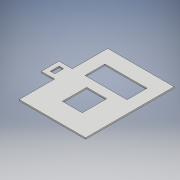
# Autodesk Inventor part: depan
Saved by Autodesk Inventor 2017 (Build 210142000, 142)
## iProperties
Created: 2017-01-06
Part Number: depan
Material: Generic
Document SubType Name: Modeling
Designer: Ghesa Bhakti
Density: 1 g/cm^3
Appearance: Default
Author: Ghesa Bhakti
Autodesk Inventor part; units mm, degrees
ref_plane "YZ Plane" through (0, 0, 0) normal (1, 0, 0) x (0, 1, 0)
ref_plane "XZ Plane" through (0, 0, 0) normal (0, 1, 0) x (-1, 0, 0)
ref_plane "XY Plane" through (0, 0, 0) normal (0, 0, 1) x (1, 0, 0)
sketch "Sketch1" plane through (0, 0, 0) normal (0, 0, 1) x (1, 0, 0)
  line L0 (27.5, 166.3577) -> (122.5, 166.3577)
  line L1 (122.5, 166.3577) -> (122.5, 121.3577)
  line L2 (122.5, 121.3577) -> (27.5, 121.3577)
  line L3 (27.5, 121.3577) -> (27.5, 166.3577)
  line L4 (52.5, 100.1) -> (97.5, 100.1)
  line L5 (97.5, 100.1) -> (97.5, 45.1)
  line L6 (97.5, 45.1) -> (52.5, 45.1)
  line L7 (52.5, 45.1) -> (52.5, 100.1)
  line L8 (0, 0) -> (150, 0)
  line L9 (0, 200) -> (150, 200)
  line L10 (0, 153.4) -> (0, 120)
  line L11 (0, 80) -> (0, 0)
  line L12 (0, 153.4) -> (0, 200)
  line L13 (0, 120) -> (-30, 120)
  line L14 (-30, 120) -> (-30, 80)
  line L15 (-30, 80) -> (0, 80)
  line L16 (-20, 110) -> (-10, 110)
  line L17 (-10, 110) -> (-10, 90)
  line L18 (-10, 90) -> (-20, 90)
  line L19 (-20, 90) -> (-20, 110)
  line L20 (150, 200) -> (150, 0)
  dimension "d0" = 150
  dimension "d49" = 200
  dimension "d50" = 40
  dimension "d51" = 80
  dimension "d52" = 10
  dimension "d53" = 95
  dimension "d54" = 45
  dimension "d55" = 45
  dimension "d56" = 55
  constraints: 42 end point, 8 perpendicular, 7 parallel, 5 horizontal, 1 vertical
  measures "d0" distance of L9.end L9.start
  measures "d49" distance of L9.end L8.end
  measures "d50" distance of L13.end L14.end
  measures "d51" distance of L11.start L8.start
  measures "d52" distance between parallel lines of L15 L18
  measures "d53" distance of L0.start L0.end
  measures "d54" distance of L0.end L1.end
  measures "d55" distance of L4.start L4.end
  measures "d56" distance of L4.end L5.end
extrude "Extrusion1" add sketch "Sketch1" along normal blind 3 contours L11 L15 L14 L13 L10 L12 L9 L20 L8 | L16 L17 L18 L19
sketch "Sketch2" plane through (0, 0, 3) normal (0, 0, 1) x (1, 0, 0)
  line L0 (-30, 80.2736) -> (0, 80.2736)
  line L1 (-20, 110.2736) -> (-10, 110.2736)
  line L2 (-10, 110.2736) -> (-10, 90.2736)
  line L3 (-10, 90.2736) -> (-20, 90.2736)
  line L4 (-20, 90.2736) -> (-20, 110.2736)
  line L5 (0, 117.7458) -> (0, 120.2736)
  point P0 (0, 0)
  constraints: 12 end point, 2 parallel, 1 horizontal, 1 perpendicular
extrude "Extrusion2" cut sketch "Sketch2" against normal blind 3
body "Solid1"
